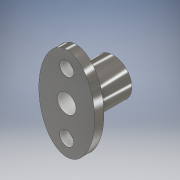
# Autodesk Inventor part: reverse gear blands
Saved by Autodesk Inventor 2017 (Build 210142000, 142)
## iProperties
Created: 2018-11-02
Part Number: reverse gear blands
Material: Generic
Document SubType Name: Modeling
Designer: User
Density: 1 g/cm^3
Appearance: Default
Author: User
Autodesk Inventor part; units mm, degrees
ref_plane "YZ Plane" through (0, 0, 0) normal (1, 0, 0) x (0, 1, 0)
ref_plane "XZ Plane" through (0, 0, 0) normal (0, 1, 0) x (-1, 0, 0)
ref_plane "XY Plane" through (0, 0, 0) normal (0, 0, 1) x (1, 0, 0)
sketch "Sketch3" plane through (0, 0, 0) normal (0, 1, 0) x (-1, 0, 0)
  ellipse E0 centre (0, 0) end of major axis (0, -10) minor radius 6
  circle A0 centre (0, 0) radius 2
  circle A1 centre (0, 6.5026) radius 1.5
  circle A2 centre (0, -6.5) radius 1.5
  dimension "d0" = 6
  dimension "d3" = 10
  dimension "d2" = 4
  dimension "d5" = 3
  dimension "d9" = 6.5026
  dimension "d11" = 3
  dimension "d12" = 6.5
  constraints: 3 centre point, 1 coincident, 2 other
  measures "d2" diameter of A0
  measures "d5" diameter of A1
  measures "d9" distance of point (0, 0) A1.centre
  measures "d11" diameter of A2
  measures "d12" distance of point (0, 0) A2.centre
extrude "Extrusion1" add sketch "Sketch3" along normal blind 2
sketch "Sketch4" plane through (0, 2, 0) normal (0, 1, 0) x (1, 0, 0)
  circle A0 centre (0, 0) radius 4
  circle A1 centre (0, 0) radius 2
  dimension "d15" = 8
  dimension "d16" = 4
  constraints: 2 centre point, 2 coincident
  measures "d15" diameter of A0
  measures "d16" diameter of A1
extrude "Extrusion2" add sketch "Sketch4" along normal blind 8
body "Solid1"
